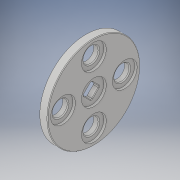
# Autodesk Inventor part: gear_collar
Saved by Autodesk Inventor 2019 (Build 230136000, 136)
## iProperties
Created: 2019-01-24
Part Number: gear_collar
Material: Generic
Document SubType Name: Modeling
Designer: Varga Daniel
Density: 1 g/cm^3
Appearance: Default
Author: Varga Daniel
Autodesk Inventor part; units mm, degrees
ref_plane "YZ Plane" through (0, 0, 0) normal (1, 0, 0) x (0, 1, 0)
ref_plane "XZ Plane" through (0, 0, 0) normal (0, 1, 0) x (-1, 0, 0)
ref_plane "XY Plane" through (0, 0, 0) normal (0, 0, 1) x (1, 0, 0)
sketch "Sketch1" plane through (0, 0, 0) normal (1, 0, 0) x (0, 1, 0)
  circle A0 centre (0, 0) radius 15
  dimension "d0" = 30
  constraints: 1 centre point, 1 coincident
  measures "d0" diameter of A0
extrude "Extrusion1" add sketch "Sketch1" along normal blind 2.5
sketch "Sketch2" plane through (2.5, 0, 0) normal (1, 0, 0) x (0, 0, -1)
  circle A0 centre (0, 0) radius 15 construction
  line L0 (-0.2828, -2.3335) -> (-2.3335, -0.2828)
  line L1 (-2.3335, 0.2828) -> (-0.2828, 2.3335)
  line L2 (0.2828, 2.3335) -> (2.3335, 0.2828)
  line L3 (2.3335, -0.2828) -> (0.2828, -2.3335)
  line L4 (0, -2.6163) -> (0, 2.6163) construction
  line L5 (-2.6163, 0) -> (2.6163, 0) construction
  arc A1 (-2.3335, 0.2828) -> (-2.3335, -0.2828) centre (-2.0506, 0) ccw
  arc A2 (-0.2828, -2.3335) -> (0.2828, -2.3335) centre (0, -2.0506) ccw
  arc A3 (2.3335, -0.2828) -> (2.3335, 0.2828) centre (2.0506, 0) ccw
  arc A4 (0.2828, 2.3335) -> (-0.2828, 2.3335) centre (0, 2.0506) ccw
  circle A5 centre (10, 0) radius 2.45
  circle A6 centre (-10, 0) radius 2.45
  circle A7 centre (0, -10) radius 2.45
  circle A8 centre (0, 10) radius 2.45
  dimension "d3" = 3.7
  dimension "d4" = 3.7
  dimension "d5" = 0.4
  dimension "d6" = 4.9
  dimension "d7" = 4.9
  dimension "d8" = 4.9
  dimension "d9" = 4.9
  dimension "d10" = 20
  dimension "d11" = 10
  dimension "d12" = 20
  dimension "d13" = 10
  constraints: 12 end point, 12 point on line, 9 centre point, 8 point on circle, 8 tangent, 4 midpoint, 3 equal radius, 2 parallel, 1 coincident, 1 horizontal, 1 perpendicular
  measures "d3" distance of L4.end L5.end
  measures "d4" distance of L5.start L4.end
  measures "d5" radius of A1
  measures "d6" diameter of A5
  measures "d7" diameter of A6
  measures "d8" diameter of A7
  measures "d9" diameter of A8
  measures "d10" distance of A7.centre A8.centre
  measures "d11" distance from line of L5 A7.centre
  measures "d12" distance of A5.centre A6.centre
  measures "d13" distance of A0.centre A6.centre
extrude "Extrusion2" cut sketch "Sketch2" against normal through all
fillet "Fillet1" radius 0.2 1 edges at (2.5, -15, 0)
sketch "Sketch3" plane through (2.5, 0, 0) normal (1, 0, 0) x (0, 0, -1)
  circle A0 centre (-10, 0) radius 2.45 construction
  circle A1 centre (10, 0) radius 2.45 construction
  arc A2 (-2.3335, 0.2828) -> (-2.3335, -0.2828) centre (-2.0506, 0) ccw construction
  line L0 (-2.3335, 0.2828) -> (-0.2828, 2.3335) construction
  arc A3 (0.2828, 2.3335) -> (-0.2828, 2.3335) centre (0, 2.0506) ccw construction
  line L1 (0.2828, 2.3335) -> (2.3335, 0.2828) construction
  arc A4 (2.3335, -0.2828) -> (2.3335, 0.2828) centre (2.0506, 0) ccw construction
  line L2 (2.3335, -0.2828) -> (0.2828, -2.3335) construction
  arc A5 (-0.2828, -2.3335) -> (0.2828, -2.3335) centre (0, -2.0506) ccw construction
  line L3 (-0.2828, -2.3335) -> (-2.3335, -0.2828) construction
  circle A6 centre (0, 10) radius 2.45 construction
  circle A7 centre (0, -10) radius 2.45 construction
  circle A8 centre (0, 0) radius 14.8 construction
  circle A9 centre (-10, 0) radius 4
  circle A10 centre (0, 10) radius 4
  circle A11 centre (10, 0) radius 4
  circle A12 centre (0, -10) radius 4
  circle A13 centre (0, 0) radius 4
  dimension "d17" = 8
  dimension "d18" = 8
  dimension "d19" = 8
  dimension "d20" = 8
  dimension "d21" = 8
  constraints: 5 centre point, 5 coincident
  measures "d17" diameter of A9
  measures "d18" diameter of A10
  measures "d19" diameter of A11
  measures "d20" diameter of A12
  measures "d21" diameter of A13
extrude "Extrusion3" cut sketch "Sketch3" against normal blind 0.8 contours A9 | A10 | A11 | A12
fillet "Fillet2" radius 0.3 4 edges at (1.7, -10, 2.45) (1.7, 0, 12.45) (1.7, 0, -7.55) (1.7, 10, 2.45)
sketch "Sketch4" plane through (2.5, 0, 0) normal (1, 0, 0) x (0, 0, -1)
  circle A0 centre (0, 0) radius 4
  dimension "d25" = 8
  constraints: 1 centre point, 1 coincident
  measures "d25" diameter of A0
extrude "Extrusion4" cut sketch "Sketch4" against normal blind 0.8
fillet "Fillet3" radius 0.2 8 edges at (1.7, 0, 2.4506) (1.7, -1.3081, 1.3081) (1.7, -2.4506, 0) (1.7, -1.3081, -1.3081) (1.7, 0, -2.4506) (1.7, 1.3081, -1.3081) (1.7, 2.4506, 0) (1.7, 1.3081, 1.3081)
equation "\"d4\" = d3"
equation "\"d7\" = d6"
equation "\"d8\" = d6"
equation "\"d9\" = d6"
equation "\"d11\" = 0.5 * d10"
equation "\"d12\" = d10"
equation "\"d13\" = 0.5 * d12"
equation "\"d18\" = d17"
equation "\"d19\" = d17"
equation "\"d20\" = d17"
equation "\"d21\" = d17"
body "Solid1"
